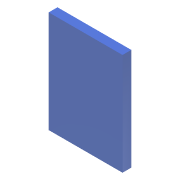
# Autodesk Inventor part: Polymer
Saved by Autodesk Inventor 2014 (Build 180170000, 170)
## iProperties
Created: 2014-09-04
Part Number: Polymer
Material: Generic
Document SubType Name: Modeling
Designer: Peele
Density: 1 g/cm^3
Appearance: Clear - Blue
Author: Peele
Autodesk Inventor part; units mm, degrees
ref_plane "YZ Plane" through (0, 0, 0) normal (1, 0, 0) x (0, 1, 0)
ref_plane "XZ Plane" through (0, 0, 0) normal (0, 1, 0) x (-1, 0, 0)
ref_plane "XY Plane" through (0, 0, 0) normal (0, 0, 1) x (1, 0, 0)
sketch "Sketch1" plane through (0, 0, 0) normal (0, 1, 0) x (-1, 0, 0)
  line L0 (-41.3704, -95.8994) -> (42.6296, -95.8994)
  line L1 (42.6296, -95.8994) -> (42.6296, 20.1006)
  line L2 (42.6296, 20.1006) -> (-41.3704, 20.1006)
  line L3 (-41.3704, 20.1006) -> (-41.3704, -95.8994)
  line L4 (-41.3704, -95.8994) -> (42.6296, 20.1006) construction
  line L5 (42.6296, -95.8994) -> (-41.3704, 20.1006) construction
  point P0 (0, 0)
  point P1 (0.6296, -37.8994)
  dimension "d0" = 84
  dimension "d1" = 116
  constraints: 12 end point, 2 midpoint, 2 parallel, 1 horizontal, 1 perpendicular
  measures "d0" distance of L1.end L2.end
  measures "d1" distance of L2.end L0.start
extrude "Extrusion1" add sketch "Sketch1" along normal blind 10
body "Solid1"
